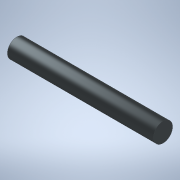
# Autodesk Inventor part: Bolt_3_23
Saved by Autodesk Inventor 2021.3 (Build 253353000, 353)
## iProperties
Created: 2021-04-16
Part Number: Bolt_3_23
Material: Iron, Cast
Document SubType Name: Modeling
Designer: domin
Density: 7.15 g/cm^3
Appearance: Iron Gray
Mass: 1.16243 g
Surface Area: 2.30907 cm^2
Volume: 0.162577 cm^3
Author: domin
Autodesk Inventor part; units mm, degrees
ref_plane "YZ Plane" through (0, 0, 0) normal (1, 0, 0) x (0, 1, 0)
ref_plane "XZ Plane" through (0, 0, 0) normal (0, 1, 0) x (-1, 0, 0)
ref_plane "XY Plane" through (0, 0, 0) normal (0, 0, 1) x (1, 0, 0)
sketch "Sketch1" plane through (0, 0, 0) normal (0, 0, 1) x (1, 0, 0)
  line L0 (0, 0) -> (23, 0)
  line L1 (23, 0) -> (23, 1.5)
  line L2 (23, 1.5) -> (0, 1.5)
  line L3 (0, 1.5) -> (0, 0)
  dimension "d0" = 23
  dimension "d1" = 1.5
  constraints: 8 end point, 2 parallel, 1 horizontal, 1 perpendicular
  measures "d0" distance of L2.end L1.end
  measures "d1" distance of L1.end L0.end
revolve "Revolution1" add sketch "Sketch1" angle 360 about axis through (0, 0, 0) along (1, 0, 0)
body "Solid1"
